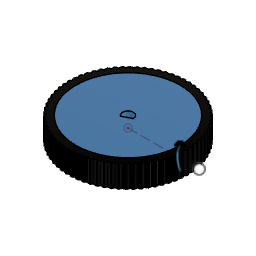
Car v6 (Autodesk Fusion 360 archive; units mm, degrees)
design "Wheel"
Autodesk Fusion 360 part; units mm, degrees
sketch "Sketch1" plane through (0, 0, 0) normal (0, 0, 1) x (1, 0, 0)
  circle A0 centre (0, 0) radius 20
  circle A1 centre (0, 0) radius 17.5
  circle A2 centre (0, 0) radius 1.8
  line L0 (0, 0) -> (-0.8104, 1.6072) construction
  line L1 (-0.8104, 1.6072) -> (0.4052, -0.8036) construction
  line L2 (0.4052, -0.8036) -> (1.7971, -0.1018) construction
  line L3 (1.7971, -0.1018) -> (-0.9867, -1.5055)
  line L4 (-0.7337, 19.9865) -> (0, 19.5)
  line L5 (0, 19.5) -> (0.7337, 19.9865)
  line L6 (-1.748, 19.4215) -> (-1.0608, 19.9718)
  line L7 (-2.5223, 19.8403) -> (-1.748, 19.4215)
  line L8 (-3.4819, 19.1866) -> (-2.8468, 19.7964)
  line L9 (-4.2906, 19.5343) -> (-3.4819, 19.1866)
  line L10 (-5.1877, 18.7973) -> (-4.6099, 19.4615)
  line L11 (-6.0244, 19.0711) -> (-5.1877, 18.7973)
  line L12 (-6.8518, 18.2566) -> (-6.3359, 18.9699)
  line L13 (-7.7097, 18.4543) -> (-6.8518, 18.2566)
  line L14 (-8.4607, 17.5689) -> (-8.0108, 18.3256)
  line L15 (-9.3329, 17.6889) -> (-8.4607, 17.5689)
  line L16 (-10.0015, 16.7398) -> (-9.6212, 17.5337)
  line L17 (-10.8809, 16.7811) -> (-10.0015, 16.7398)
  line L18 (-11.4618, 15.7758) -> (-11.1542, 16.6007)
  line L19 (-12.3414, 15.7382) -> (-11.4618, 15.7758)
  line L20 (-12.8298, 14.6849) -> (-12.5974, 15.534)
  line L21 (-13.7024, 14.5686) -> (-12.8298, 14.6849)
  line L22 (-14.0945, 13.4757) -> (-13.9391, 14.3423)
  line L23 (-14.9532, 13.2816) -> (-14.0945, 13.4757)
  line L24 (-15.2457, 12.1581) -> (-15.1687, 13.035)
  line L25 (-16.0836, 11.8878) -> (-15.2457, 12.1581)
  line L26 (-16.2742, 10.7425) -> (-16.276, 11.6228)
  line L27 (-17.0844, 10.3982) -> (-16.2742, 10.7425)
  line L28 (-17.1716, 9.2404) -> (-17.2524, 10.1171)
  line L29 (-17.9477, 8.8249) -> (-17.1716, 9.2404)
  line L30 (-17.9308, 7.664) -> (-18.0898, 8.5299)
  line L31 (-18.6665, 7.1806) -> (-17.9308, 7.664)
  line L32 (-18.5456, 6.0258) -> (-18.7816, 6.874)
  line L33 (-19.2351, 5.4784) -> (-18.5456, 6.0258)
  line L34 (-19.0111, 4.3392) -> (-19.3222, 5.1627)
  line L35 (-19.6487, 3.7321) -> (-19.0111, 4.3392)
  line L36 (-19.3235, 2.6175) -> (-19.7072, 3.4099)
  line L37 (-19.9041, 1.9558) -> (-19.3235, 2.6175)
  line L38 (-19.4804, 0.8749) -> (-19.9335, 1.6297)
  line L39 (-19.9993, 0.1637) -> (-19.4804, 0.8749)
  line L40 (-19.4804, -0.8749) -> (-19.9993, -0.1637)
  line L41 (-19.9335, -1.6297) -> (-19.4804, -0.8749)
  line L42 (-19.3235, -2.6175) -> (-19.9041, -1.9558)
  line L43 (-19.7072, -3.4099) -> (-19.3235, -2.6175)
  line L44 (-19.0111, -4.3392) -> (-19.6487, -3.7321)
  line L45 (-19.3222, -5.1627) -> (-19.0111, -4.3392)
  line L46 (-18.5456, -6.0258) -> (-19.2351, -5.4784)
  line L47 (-18.7816, -6.874) -> (-18.5456, -6.0258)
  line L48 (-17.9308, -7.664) -> (-18.6665, -7.1806)
  line L49 (-18.0898, -8.5299) -> (-17.9308, -7.664)
  line L50 (-17.1716, -9.2404) -> (-17.9477, -8.8249)
  line L51 (-17.2524, -10.1171) -> (-17.1716, -9.2404)
  line L52 (-16.2742, -10.7425) -> (-17.0844, -10.3982)
  line L53 (-16.276, -11.6228) -> (-16.2742, -10.7425)
  line L54 (-15.2457, -12.1581) -> (-16.0836, -11.8878)
  line L55 (-15.1687, -13.035) -> (-15.2457, -12.1581)
  line L56 (-14.0945, -13.4757) -> (-14.9532, -13.2816)
  line L57 (-13.9391, -14.3423) -> (-14.0945, -13.4757)
  line L58 (-12.8298, -14.6849) -> (-13.7024, -14.5686)
  line L59 (-12.5974, -15.534) -> (-12.8298, -14.6849)
  line L60 (-11.4618, -15.7758) -> (-12.3414, -15.7382)
  line L61 (-11.1542, -16.6007) -> (-11.4618, -15.7758)
  line L62 (-10.0015, -16.7398) -> (-10.8809, -16.7811)
  line L63 (-9.6212, -17.5337) -> (-10.0015, -16.7398)
  line L64 (-8.4607, -17.5689) -> (-9.3329, -17.6889)
  line L65 (-8.0108, -18.3256) -> (-8.4607, -17.5689)
  line L66 (-6.8518, -18.2566) -> (-7.7097, -18.4543)
  line L67 (-6.3359, -18.9699) -> (-6.8518, -18.2566)
  line L68 (-5.1877, -18.7973) -> (-6.0244, -19.0711)
  line L69 (-4.6099, -19.4615) -> (-5.1877, -18.7973)
  line L70 (-3.4819, -19.1866) -> (-4.2906, -19.5343)
  line L71 (-2.8468, -19.7964) -> (-3.4819, -19.1866)
  line L72 (-1.748, -19.4215) -> (-2.5223, -19.8403)
  line L73 (-1.0608, -19.9718) -> (-1.748, -19.4215)
  line L74 (0, -19.5) -> (-0.7337, -19.9865)
  line L75 (0.7337, -19.9865) -> (0, -19.5)
  line L76 (1.748, -19.4215) -> (1.0608, -19.9718)
  line L77 (2.5223, -19.8403) -> (1.748, -19.4215)
  line L78 (3.4819, -19.1866) -> (2.8468, -19.7964)
  line L79 (4.2906, -19.5343) -> (3.4819, -19.1866)
  line L80 (5.1877, -18.7973) -> (4.6099, -19.4615)
  line L81 (6.0244, -19.0711) -> (5.1877, -18.7973)
  line L82 (6.8518, -18.2566) -> (6.3359, -18.9699)
  line L83 (7.7097, -18.4543) -> (6.8518, -18.2566)
  line L84 (8.4607, -17.5689) -> (8.0108, -18.3256)
  line L85 (9.3329, -17.6889) -> (8.4607, -17.5689)
  line L86 (10.0015, -16.7398) -> (9.6212, -17.5337)
  line L87 (10.8809, -16.7811) -> (10.0015, -16.7398)
  line L88 (11.4618, -15.7758) -> (11.1542, -16.6007)
  line L89 (12.3414, -15.7382) -> (11.4618, -15.7758)
  line L90 (12.8298, -14.6849) -> (12.5974, -15.534)
  line L91 (13.7024, -14.5686) -> (12.8298, -14.6849)
  line L92 (14.0945, -13.4757) -> (13.9391, -14.3423)
  line L93 (14.9532, -13.2816) -> (14.0945, -13.4757)
  line L94 (15.2457, -12.1581) -> (15.1687, -13.035)
  line L95 (16.0836, -11.8878) -> (15.2457, -12.1581)
  line L96 (16.2742, -10.7425) -> (16.276, -11.6228)
  line L97 (17.0844, -10.3982) -> (16.2742, -10.7425)
  line L98 (17.1716, -9.2404) -> (17.2524, -10.1171)
  line L99 (17.9477, -8.8249) -> (17.1716, -9.2404)
  line L100 (17.9308, -7.664) -> (18.0898, -8.5299)
  line L101 (18.6665, -7.1806) -> (17.9308, -7.664)
  line L102 (18.5456, -6.0258) -> (18.7816, -6.874)
  line L103 (19.2351, -5.4784) -> (18.5456, -6.0258)
  line L104 (19.0111, -4.3392) -> (19.3222, -5.1627)
  line L105 (19.6487, -3.7321) -> (19.0111, -4.3392)
  line L106 (19.3235, -2.6175) -> (19.7072, -3.4099)
  line L107 (19.9041, -1.9558) -> (19.3235, -2.6175)
  line L108 (19.4804, -0.8749) -> (19.9335, -1.6297)
  line L109 (19.9993, -0.1637) -> (19.4804, -0.8749)
  line L110 (19.4804, 0.8749) -> (19.9993, 0.1637)
  line L111 (19.9335, 1.6297) -> (19.4804, 0.8749)
  line L112 (19.3235, 2.6175) -> (19.9041, 1.9558)
  line L113 (19.7072, 3.4099) -> (19.3235, 2.6175)
  line L114 (19.0111, 4.3392) -> (19.6487, 3.7321)
  line L115 (19.3222, 5.1627) -> (19.0111, 4.3392)
  line L116 (18.5456, 6.0258) -> (19.2351, 5.4784)
  line L117 (18.7816, 6.874) -> (18.5456, 6.0258)
  line L118 (17.9308, 7.664) -> (18.6665, 7.1806)
  line L119 (18.0898, 8.5299) -> (17.9308, 7.664)
  line L120 (17.1716, 9.2404) -> (17.9477, 8.8249)
  line L121 (17.2524, 10.1171) -> (17.1716, 9.2404)
  line L122 (16.2742, 10.7425) -> (17.0844, 10.3982)
  line L123 (16.276, 11.6228) -> (16.2742, 10.7425)
  line L124 (15.2457, 12.1581) -> (16.0836, 11.8878)
  line L125 (15.1687, 13.035) -> (15.2457, 12.1581)
  line L126 (14.0945, 13.4757) -> (14.9532, 13.2816)
  line L127 (13.9391, 14.3423) -> (14.0945, 13.4757)
  line L128 (12.8298, 14.6849) -> (13.7024, 14.5686)
  line L129 (12.5974, 15.534) -> (12.8298, 14.6849)
  line L130 (11.4618, 15.7758) -> (12.3414, 15.7382)
  line L131 (11.1542, 16.6007) -> (11.4618, 15.7758)
  line L132 (10.0015, 16.7398) -> (10.8809, 16.7811)
  line L133 (9.6212, 17.5337) -> (10.0015, 16.7398)
  line L134 (8.4607, 17.5689) -> (9.3329, 17.6889)
  line L135 (8.0108, 18.3256) -> (8.4607, 17.5689)
  line L136 (6.8518, 18.2566) -> (7.7097, 18.4543)
  line L137 (6.3359, 18.9699) -> (6.8518, 18.2566)
  line L138 (5.1877, 18.7973) -> (6.0244, 19.0711)
  line L139 (4.6099, 19.4615) -> (5.1877, 18.7973)
  line L140 (3.4819, 19.1866) -> (4.2906, 19.5343)
  line L141 (2.8468, 19.7964) -> (3.4819, 19.1866)
  line L142 (1.748, 19.4215) -> (2.5223, 19.8403)
  line L143 (1.0608, 19.9718) -> (1.748, 19.4215)
  dimension "d1" = 40
  dimension "d2" = 35
  dimension "d3" = 3.6
  dimension "d4" = 2.7
  dimension "d6" = 360
  constraint coincident A0.centre A1.centre
  constraint concentric A0 A1
  constraint coincident A2 L0.end
  constraint parallel L0 L1
  constraint coincident A2 L2.end
  constraint perpendicular L1 L2
  constraint coincident A2 L3.end
  constraint parallel L2 L3
  constraint coincident A0 L4.start
  constraint coincident A0 L5.end
  measures "d1" diameter of A0
  measures "d2" diameter of A1
  measures "d3" diameter of A2
  measures "d4" distance of L0.end L1.end
extrude "Extrude1" add sketch "Sketch1" along normal mid plane 7.4 contours A1 | A2 L3 picked at (0.1038, -1.1122) makes body 1
extrude "Extrude2" add sketch "Sketch1" along normal mid plane 7.4 separate body contours A0 L4 L5 L6 L7 L8 L9 L10 L11 L12 L13 L14 L15 L16 L17 L18 L19 L20 L21 L22 L23 L24 L25 L26 L27 L28 L29 L30 L31 L32 L33 L34 L35 L36 L37 L38 L39 L40 L41 L42 L43 L44 L45 L46 L47 L48 L49 L50 L51 L52 L53 L54 L55 L56 L57 L58 L59 L60 L61 L62 L63 L64 L65 L66 L67 L68 L69 L70 L71 L72 L73 L74 L75 L76 L77 L78 L79 L80 L81 L82 L83 L84 L85 L86 L87 L88 L89 L90 L91 L92 L93 L94 L95 L96 L97 L98 L99 L100 L101 L102 L103 L104 L105 L106 L107 L108 L109 L110 L111 L112 L113 L114 L115 L116 L117 L118 L119 L120 L121 L122 L123 L124 L125 L126 L127 L128 L129 L130 L131 L132 L133 L134 L135 L136 L137 L138 L139 L140 L141 L142 L143 makes body 2
sketch "Sketch2" plane through (0, 0, 0) normal (0, 1, 0) x (1, 0, 0)
  line L0 (0, 0) -> (17.5, 0)
  line L1 (17.5, 0) -> (17.5, -3.7)
  line L2 (17.5, 0) -> (17.5, 3.7)
  arc A0 (17.5, 3.7) -> (17.5, -3.7) centre (23.845, 0) ccw
  line L3 (17.5, 3.7) -> (17.5, 3.4) construction
  arc A1 (17.5, 3.4) -> (17.5, -3.4) centre (23.9228, 0) ccw
  point P0 (17.5, -3.4)
  dimension "d11" = 17.5
  dimension "d12" = 3.7
  dimension "d13" = 3.7
  dimension "d15" = 0.3
  constraint coincident L0.start origin
  constraint horizontal L0
  constraint perpendicular L0 L1
  constraint perpendicular L0 L2
  constraint parallel L2 L3
  constraint symmetric L0 L3.end P0
  constraint tangent A0 A1
  constraint coincident P0 A1.end
  measures "d11" distance of L0.start L0.end
  measures "d12" distance of L0.end L1.end
  measures "d13" distance of L0.end L2.end
  measures "d15" distance of L2.end L3.end
revolve "Revolve1" cut sketch "Sketch2" angle 360 about axis through (0, 0, 1.75) along (0, 0, 1) bodies 1
revolve "Revolve2" add sketch "Sketch2" angle 360 about axis through (0, 0, -7.4) along (0, 0, 1) contours L0 L2 A1 | L0 L1 A1 bodies 2
equation "d11 = ( 35 / 2 ) * 1 mm"
